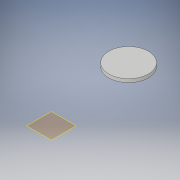
# Autodesk Inventor part: Geschwindigkeitsschild_Teil_Oben
Saved by Autodesk Inventor 2019.5 (Build 235369000, 369)
## iProperties
Created: 2021-09-30
Part Number: Geschwindigkeitsschild_Teil_Oben
Material: Generisch
Document SubType Name: Modeling
Designer: mritt
Density: 1 g/cm^3
Appearance: Vorgabe
Author: mritt
Autodesk Inventor part; units mm, degrees
ref_plane "YZ Plane" through (0, 0, 0) normal (1, 0, 0) x (0, 1, 0)
ref_plane "XZ Plane" through (0, 0, 0) normal (0, 1, 0) x (-1, 0, 0)
ref_plane "XY Plane" through (0, 0, 0) normal (0, 0, 1) x (1, 0, 0)
ref_plane "Arbeitsebene1" through (0, 3, 0) normal (0, 1, 0) x (1, 0, 0)
sketch "Skizze7" plane through (0, 3, 0) normal (0, 1, 0) x (1, 0, 0)
  circle A0 centre (-11.3272, 79.8082) radius 17.5
  point P0 (0, 0)
  dimension "d23" = 35
  constraints: 1 centre point
  measures "d23" diameter of A0
extrude "Extrusion6" add sketch "Skizze7" along normal blind 3
